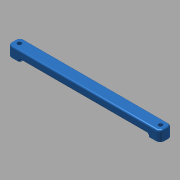
# Autodesk Inventor part: BatteryHolderTopStrap
Saved by Autodesk Inventor 2014 (Build 180170000, 170)
## iProperties
Created: 2014-10-22
Part Number: BatteryHolderTopStrap
Material: Generic
Document SubType Name: Modeling
Designer: Karl
Density: 1 g/cm^3
Appearance: Cyan
Author: Karl
Autodesk Inventor part; units mm, degrees
ref_plane "YZ Plane" through (0, 0, 0) normal (1, 0, 0) x (0, 1, 0)
ref_plane "XZ Plane" through (0, 0, 0) normal (0, 1, 0) x (-1, 0, 0)
ref_plane "XY Plane" through (0, 0, 0) normal (0, 0, 1) x (1, 0, 0)
sketch "Sketch1" plane through (0, 0, 0) normal (0, 1, 0) x (-1, 0, 0)
  line L0 (-59.69, 4.7625) -> (59.69, 4.7625)
  line L1 (59.69, 4.7625) -> (59.69, -4.7625)
  line L2 (59.69, -4.7625) -> (-59.69, -4.7625)
  line L3 (-59.69, -4.7625) -> (-59.69, 4.7625)
  point P0 (0, 0)
  point P1 (0, 4.7625)
  point P2 (-59.69, 0)
  dimension "d0" = 119.38
  dimension "d1" = 9.525
  constraints: 8 end point, 2 midpoint, 2 parallel, 1 horizontal, 1 horizontal alignment, 1 perpendicular, 1 vertical alignment
  measures "d0" distance of L0.start L0.end
  measures "d1" distance of L2.end L0.start
extrude "Extrusion1" add sketch "Sketch1" along normal blind 6.35
sketch "Sketch2" plane through (0, 6.35, 0) normal (0, 1, 0) x (1, 0, 0)
  point P0 (0, 0)
  point P1 (-55.245, 0)
  point P2 (55.245, 0)
  dimension "d4" = 55.245
  dimension "d5" = 55.245
  measures "d4" distance of point (55.245, 0) point (0, 0)
  measures "d5" distance of point (0, 0) point (-55.245, 0)
hole "Hole1" at (-55.245, 6.35, 0) at (55.245, 6.35, 0) direction (0, -1, 0) diameter 3.302 depth 25.4 tip angle 118
fillet "Fillet1" radius 3.175 4 edges at (-59.69, 3.175, 4.7625) (-59.69, 3.175, -4.7625) (59.69, 3.175, 4.7625) (59.69, 3.175, -4.7625)
fillet "Fillet2" radius 1.27 8 edges at (58.7601, 6.35, 3.8326) (59.69, 6.35, 0) (58.7601, 6.35, -3.8326) (0, 6.35, -4.7625) (-58.7601, 6.35, -3.8326) (-59.69, 6.35, 0) (-58.7601, 6.35, 3.8326) (0, 6.35, 4.7625)
sketch "Sketch3" plane through (0, 0, 0) normal (0, -1, 0) x (1, 0, 0)
  arc A0 (56.515, -4.7625) -> (59.69, -1.5875) centre (56.515, -1.5875) ccw projected
  line L0 (59.69, -1.5875) -> (59.69, 1.5875) projected
  arc A1 (59.69, 1.5875) -> (56.515, 4.7625) centre (56.515, 1.5875) ccw projected
  line L1 (56.515, 4.7625) -> (-56.515, 4.7625) projected
  arc A2 (-56.515, 4.7625) -> (-59.69, 1.5875) centre (-56.515, 1.5875) ccw projected
  line L2 (-59.69, 1.5875) -> (-59.69, -1.5875) projected
  arc A3 (-59.69, -1.5875) -> (-56.515, -4.7625) centre (-56.515, -1.5875) ccw projected
  line L3 (-56.515, -4.7625) -> (56.515, -4.7625) projected
  circle A4 centre (-55.245, 0) radius 1.651 projected
  circle A5 centre (55.245, 0) radius 1.651 projected
  line L4 (-50.165, 4.7625) -> (-50.165, -4.7625)
  line L5 (50.165, 4.7625) -> (50.165, -4.7625)
  point P0 (0, 0)
  dimension "d15" = 9.525
  dimension "d16" = 9.525
  constraints: 4 end point, 4 point on line, 2 perpendicular
  measures "d15" distance between parallel lines of L4 L2
  measures "d16" distance between parallel lines of L0 L5
extrude "Extrusion2" add sketch "Sketch3" along normal blind 1.651 contours L3 L5 L1 A1 L0 A0 | L3 A3 L2 A2 L1 L4
fillet "Fillet3" radius 1.27 8 edges at (0, 0, 4.7625) (-50.165, -0.8255, 4.7625) (-50.165, -0.8255, -4.7625) (-50.165, 0, 0) (0, 0, -4.7625) (50.165, -0.8255, 4.7625) (50.165, 0, 0) (50.165, -0.8255, -4.7625)
body "Solid1"
